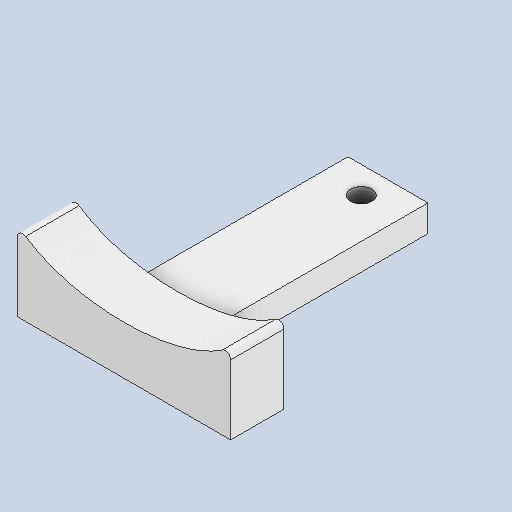
# Autodesk Inventor part: Part 1 menton
Saved by Autodesk Inventor 2023 (Build 270158000, 158)
## iProperties
Created: 2022-10-28
Part Number: Part 1 menton
Material: ABS Plastic
Document SubType Name: Modeling
Designer: Lenovo
Density: 1.06 g/cm^3
Appearance: Smooth - White
Author: Lenovo
Autodesk Inventor part; units mm, degrees
ref_plane "YZ Plane" through (0, 0, 0) normal (1, 0, 0) x (0, 1, 0)
ref_plane "XZ Plane" through (0, 0, 0) normal (0, 1, 0) x (-1, 0, 0)
ref_plane "XY Plane" through (0, 0, 0) normal (0, 0, 1) x (1, 0, 0)
sketch "Sketch3" plane through (0, 0, 0) normal (0, 0, 1) x (1, 0, 0)
  line L0 (0, 0) -> (80, 0)
  line L1 (80, 0) -> (80, -30)
  line L2 (80, -30) -> (0, -30)
  line L3 (0, -30) -> (0, 0)
  line L4 (0, 0) -> (14.7083, -12.3417) construction
  line L5 (14.7083, -12.3417) -> (40, -15) construction
  line L6 (40, -15) -> (65.2917, -12.3417) construction
  line L7 (65.2917, -12.3417) -> (80, 0) construction
  spline S0 degree 4 poles (0, 0) (14.7083, -12.3417) (40, -15) (65.2917, -12.3417) (80, 0) knots 1 1 1 1 1 2 2 2 2 2
  point P0 (52.6458, -13.6709)
  dimension "d13" = 80
  dimension "d14" = 30
  dimension "d15" = 15
  dimension "d16" = 40
  dimension "d17" = 50
  dimension "d18" = 50
  dimension "d19" = 6
  dimension "d21" = 6
  constraints: 8 end point, 2 parallel, 1 horizontal, 1 midpoint, 1 perpendicular, 3 other
  measures "d13" distance of L1.end L2.end
  measures "d14" distance of L0.end L1.end
  measures "d15" distance from line of L2 L5.end
  measures "d16" distance from line of L3 L5.end
  measures "d17" angle of L1 L7
  measures "d18" angle of L3 L4
  measures "d19" angle of L2 L5
  measures "d21" angle of L2 L6
extrude "Extrusion1" add sketch "Sketch3" along normal blind 20 contours S0 L1 L2 L3
sketch "Sketch4" plane through (0, 0, 0) normal (0, 0, -1) x (-1, 0, 0)
  line L0 (-25, -25) -> (-55, -25)
  line L1 (-55, -25) -> (-55, -15)
  line L2 (-55, -15) -> (-25, -15)
  line L3 (-25, -15) -> (-25, -25)
  line L4 (-40, -25) -> (-40, -15) construction
  line L5 (-80, -30) -> (-80, 0) projected
  line L6 (0, -30) -> (-80, -30) projected
  point P0 (0, 0)
  dimension "d24" = 30
  dimension "d25" = 40
  dimension "d26" = 5
  dimension "d27" = 10
  constraints: 10 end point, 2 midpoint, 2 parallel, 1 horizontal, 1 perpendicular
  measures "d24" distance of L0.start L0.end
  measures "d25" distance between parallel lines of L5 L4
  measures "d26" distance between parallel lines of L6 L0
  measures "d27" distance of L0.end L1.end
extrude "Extrusion2" add sketch "Sketch4" along normal blind 80
sketch "Sketch7" plane through (25, -15, 0) normal (0, 1, 0) x (1, 0, 0)
  line L0 (0, 55) -> (20, 55)
  line L1 (20, 55) -> (20, 75)
  line L2 (20, 75) -> (0, 75)
  line L3 (0, 75) -> (0, 55)
  line L4 (30, 0) -> (0, 0) projected
  line L5 (30, 0) -> (30, 80) projected
  line L6 (0, 80) -> (30, 80) projected
  line L7 (0, 0) -> (0, 80) projected
  circle A0 centre (10, 65) radius 4
  line L8 (0, 55) -> (0, 55)
  line L9 (0, 0) -> (0, 80) projected
  line L10 (20, 55) -> (30, 55)
  point P0 (-25, 0)
  point P1 (20, 65)
  point P2 (10, 75)
  point P3 (0, 35)
  dimension "d40" = 10
  dimension "d42" = 20
  dimension "d43" = 20
  dimension "d44" = 8
  dimension "d51" = 15
  constraints: 12 end point, 3 point on line, 2 midpoint, 2 parallel, 2 perpendicular, 1 centre point, 1 horizontal, 1 horizontal alignment, 1 vertical alignment
  measures "d40" distance between parallel lines of L5 L1
  measures "d42" distance from line of point (20, 65) L3
  measures "d43" distance between parallel lines of L0 L2
  measures "d44" diameter of A0
  measures "d51" distance from line of L6 A0.centre
extrude "Extrusion4" add sketch "Sketch7" along normal blind 10 contours L3 L2 L1 L0 | L1 L2 L7 L6 L5 L10 | A0
sketch "Sketch9" plane through (0, 0, -80) normal (0, 0, -1) x (-1, 0, 0)
  line L0 (-55, -25) -> (-55, -5) projected
  line L1 (-55, -25) -> (-25, -25) projected
  line L2 (-25, -25) -> (-25, -5) projected
  line L3 (-55, -5) -> (-25, -5) projected
  point P0 (0, 0)
extrude "Extrusion7" cut sketch "Sketch9" against normal blind 19
sketch "Sketch10" plane through (0, 0, -61) normal (0, 0, -1) x (-1, 0, 0)
  line L0 (-40, -5) -> (-40, -25) construction
  line L1 (-25, -5) -> (-55, -5) projected
  line L2 (-25, -25) -> (-55, -25) projected
  line L3 (-55, -5) -> (-25, -5)
  line L4 (-25, -5) -> (-25, -25)
  line L5 (-25, -25) -> (-55, -25)
  line L6 (-55, -25) -> (-55, -5)
  line L7 (-55, -25) -> (-55, -5) projected
  line L8 (-25, -5) -> (-25, -25) projected
  line L9 (-55, -15) -> (-25, -15)
  line L10 (-25, -15) -> (-25, -25)
  line L11 (-25, -25) -> (-55, -25)
  line L12 (-55, -25) -> (-55, -15)
  point P0 (0, 0)
  dimension "d81" = 10
  constraints: 18 end point, 4 parallel, 2 horizontal, 2 midpoint, 2 perpendicular, 1 other
  measures "d81" distance between parallel lines of L2 L9
extrude "Extrusion10" add sketch "Sketch10" along normal blind 18
sketch "Sketch12" plane through (25, -5, 0) normal (0, 1, 0) x (1, 0, 0)
  line L0 (0, 79) -> (0, 55) projected
  line L1 (0, 55) -> (30, 55) projected
  line L2 (30, 55) -> (30, 79) projected
  line L3 (0, 79) -> (30, 79) projected
  line L4 (0, 0) -> (0, 79) projected
  line L5 (30, 0) -> (30, 79) projected
  line L6 (0, 79) -> (30, 79)
  line L7 (30, 79) -> (30, 64)
  line L8 (30, 64) -> (0, 64)
  line L9 (0, 64) -> (0, 79)
  point P0 (-25, 0)
  point P1 (0, 64)
  dimension "d84" = 15
  constraints: 8 end point, 2 parallel, 1 horizontal, 1 perpendicular, 1 point on line
  measures "d84" distance between parallel lines of L3 L8
extrude "Extrusion11" cut sketch "Sketch12" against normal blind 15 contours L3 L2 L8 L0
sketch "Sketch13" plane through (25, -20, 0) normal (0, 1, 0) x (1, 0, 0)
  line L0 (30, 79) -> (30, 64) projected
  line L1 (0, 79) -> (30, 79) projected
  line L2 (0, 64) -> (0, 79) projected
  line L3 (30, 64) -> (0, 64) projected
  circle A0 centre (7, 71.5) radius 4
  circle A1 centre (23, 71.5) radius 4
  circle A2 centre (7, 71.5) radius 6
  circle A3 centre (23, 71.5) radius 6
  point P0 (-25, 0)
  point P1 (0, 71.5)
  dimension "d87" = 8
  dimension "d88" = 8
  dimension "d89" = 7.5
  dimension "d90" = 7.5
  dimension "d91" = 7
  dimension "d92" = 7
  dimension "d93" = 2
  dimension "d94" = 2
  constraints: 4 centre point, 1 midpoint
  measures "d87" diameter of A0
  measures "d88" diameter of A1
  measures "d89" distance from line of L1 A0.centre
  measures "d90" distance from line of L1 A1.centre
  measures "d91" distance of point (0, 71.5) A0.centre
  measures "d92" distance from line of L0 A1.centre
  measures "d93" radial gap between concentric circles of A0 A2
  measures "d94" radial gap between concentric circles of A1 A3
extrude "Extrusion14" add sketch "Sketch13" along normal blind 15 contours L0 L3 L2 L1 | A0 | A1 | A2 | A3
sketch "Sketch14" plane through (25, -15, 0) normal (0, 1, 0) x (1, 0, 0)
  line L0 (30, 0) -> (30, 79) projected
  line L1 (30, 55) -> (0, 55)
  line L2 (0, 55) -> (0, 39)
  line L3 (0, 39) -> (30, 39)
  line L4 (30, 39) -> (30, 55)
  line L5 (30, 55) -> (0, 55) projected
  point P0 (-25, 0)
  point P1 (30, 39)
  dimension "d101" = 30
  dimension "d102" = 16
  constraints: 8 end point, 2 parallel, 1 collinear, 1 horizontal, 1 perpendicular, 1 point on line
  measures "d101" distance of L3.end L2.end
  measures "d102" distance of L2.end L1.end
extrude "Extrusion15" add sketch "Sketch14" along normal up to surface (10 mm away)
sketch "Sketch15" plane through (25, -5, 0) normal (0, 1, 0) x (1, 0, 0)
  line L0 (30, 79) -> (0, 79) projected
  line L1 (0, 79) -> (0, 39) projected
  point P0 (-25, 0)
  point P1 (15, 69)
  dimension "d105" = 10
  dimension "d106" = 15
  measures "d105" distance from line of L0 point (15, 69)
  measures "d106" distance from line of L1 point (15, 69)
hole "Hole1" at (40, -5, -69) direction (0, -1, 0) diameter 8 depth 20
sketch "Sketch16" plane through (25, -5, 0) normal (0, 1, 0) x (1, 0, 0)
  circle A0 centre (15, 69) radius 4 projected
  line L0 (0, 79) -> (0, 39) projected
  line L1 (30, 39) -> (0, 39) projected
  line L2 (30, 79) -> (30, 39) projected
  line L3 (30, 79) -> (0, 79) projected
  point P0 (-25, 0)
extrude "Extrusion16" cut sketch "Sketch16" against normal up to surface (10 mm away)
fillet "Fillet1" radius 2 2 edges at (80, 0, 10) (0, 0, 10)
thread "Thread1" size "M8x1.25" class "6H" standard "ANSI Metric M Profile" full length
body "Solid2"
